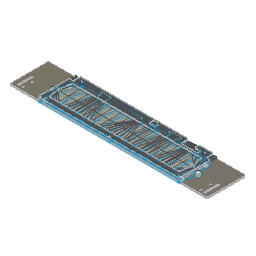
slidrr-housing (Autodesk Fusion 360 design; units mm, degrees)
part number: 2026-08-23-00-43-32-285
Autodesk Fusion 360 part; units mm, degrees
note: some values were not read from the file. Chosen so that the rebuilt part matches the saved one: which bodies a step acts on.
(part 1 of 2)
sketch "Primitive 1 (Outline + Screw Holes)" plane through (0, 0, 0) normal (0, 1, 0) x (1, 0, 0)
  line L0 (3, 0) -> (496.9999, 0)
  line L1 (499.9999, 3) -> (499.9999, 133.475)
  line L2 (496.9999, 136.475) -> (3, 136.475)
  line L3 (0, 133.475) -> (0, 3)
  arc A0 (499.9999, 133.475) -> (496.9999, 136.475) centre (496.9999, 133.475) ccw
  arc A1 (496.9999, 0) -> (499.9999, 3) centre (496.9999, 3) ccw
  arc A2 (0, 3) -> (3, 0) centre (3, 3) ccw
  arc A3 (3, 136.475) -> (0, 133.475) centre (3, 133.475) ccw
  circle A4 centre (495.2019, 4.225) radius 1.5
  circle A5 centre (250.0019, 4.225) radius 1.5
  circle A6 centre (5.0019, 4.225) radius 1.5
  circle A7 centre (6.475, 60.375) radius 1.5
  circle A8 centre (493.525, 60.375) radius 1.5
  circle A9 centre (469.2019, 123.225) radius 1.5
  circle A10 centre (31.0019, 123.225) radius 1.5
  circle A11 centre (250.0019, 117.225) radius 1.5
  point P0 (0, 136.475)
  dimension "d1" = 136.475
  dimension "d2" = 3
  dimension "d3" = 3
  dimension "d4" = 3
  dimension "d5" = 3
  dimension "d7" = 3
  dimension "d8" = 3
  dimension "d9" = 3
  dimension "d10" = 3
  dimension "d11" = 3
  constraint horizontal L0
  constraint vertical L1
  constraint horizontal L2
  constraint vertical L3
  constraint tangent L1 A0
  constraint tangent L2 A0
  constraint tangent L0 A1
  constraint tangent L1 A1
  constraint equal A0 A1
  constraint coincident origin L0
  constraint coincident origin L3
  constraint tangent L0 A2
  constraint tangent L3 A2
  constraint equal A0 A2
  constraint coincident P0 L2
  constraint coincident P0 L3
  constraint tangent L2 A3
  constraint tangent L3 A3
  constraint equal A0 A3
  measures "d1" distance of origin P0
  measures "d2" radius of A0
  measures "d3" diameter of A4
  measures "d4" diameter of A5
  measures "d5" diameter of A6
  measures "d7" diameter of A7
  measures "d8" diameter of A8
  measures "d9" diameter of A9
  measures "d10" diameter of A10
  measures "d11" diameter of A11
other "Base Mesh Feature3"
other "Modify13"
other "Modify14"
sketch "Midplate LGP" plane through (0, 0, 0) normal (0, 1, 0) x (1, 0, 0)
  line L0 (306.25, 19.35) -> (306.25, 101.35)
  arc A0 (0, 3) -> (3, 0) centre (3, 3) ccw
  line L1 (128, 106) -> (106, 106)
  line L2 (300, 128) -> (300, 118)
  line L3 (103.25, 19.35) -> (103.25, 101.35)
  arc A1 (434.5275, 124) -> (437.5275, 121) centre (437.5275, 124) ccw
  line L4 (3, 0) -> (497.0008, 0)
  line L5 (394, 136.475) -> (17, 136.475)
  line L6 (422.25, 19.35) -> (422.25, 101.35)
  line L7 (454.75, 19.35) -> (454.75, 101.35)
  line L8 (281, 131) -> (297, 131)
  arc A2 (98, 130) -> (95, 127) centre (98, 127) ccw
  arc A3 (297, 115) -> (300, 118) centre (297, 118) ccw
  arc A4 (300, 128) -> (297, 131) centre (297, 128) ccw
  line L9 (338.75, 19.35) -> (338.75, 101.35)
  line L10 (19.75, 19.35) -> (19.75, 101.35)
  arc A5 (486.0019, 133.475) -> (483.0019, 136.475) centre (483.0019, 133.475) ccw
  line L11 (434.5275, 133.475) -> (434.5275, 124)
  line L12 (278, 118) -> (278, 128)
  circle A6 centre (5.0019, 4.225) radius 1.5
  line L13 (48.75, 19.35) -> (48.75, 101.35)
  line L14 (397, 112) -> (397, 133.475)
  circle A7 centre (469.2019, 123.225) radius 1.5
  line L15 (135.75, 19.35) -> (135.75, 101.35)
  line L16 (251.75, 19.35) -> (251.75, 101.35)
  line L17 (486.0019, 114) -> (486.0019, 133.475)
  line L18 (374, 110) -> (374, 121)
  line L19 (100, 123) -> (98, 123)
  arc A8 (377, 124) -> (374, 121) centre (377, 121) ccw
  line L20 (132.25, 19.35) -> (132.25, 101.35)
  line L21 (309.75, 19.35) -> (309.75, 101.35)
  line L22 (219.25, 19.35) -> (219.25, 101.35)
  line L23 (95, 126) -> (95, 127)
  circle A9 centre (495.2019, 4.225) radius 1.5
  line L24 (193.75, 19.35) -> (193.75, 101.35)
  line L25 (437.5275, 121) -> (454, 121)
  line L26 (14, 114) -> (14, 133.475)
  line L27 (335.25, 19.35) -> (335.25, 101.35)
  arc A10 (486.0019, 114) -> (489.0019, 111) centre (489.0019, 114) ccw
  circle A11 centre (250.0019, 4.225) radius 1.5
  line L28 (222.75, 19.35) -> (222.75, 101.35)
  line L29 (77.75, 19.35) -> (77.75, 101.35)
  line L30 (451.25, 19.35) -> (451.25, 101.35)
  line L31 (457, 118) -> (457, 112)
  arc A12 (371, 107) -> (374, 110) centre (371, 110) ccw
  arc A13 (377, 124) -> (380, 127) centre (377, 127) ccw
  arc A14 (103, 109) -> (106, 106) centre (106, 109) ccw
  arc A15 (499.9999, 108) -> (496.9999, 111) centre (496.9999, 108) ccw
  circle A16 centre (6.475, 60.35) radius 1.5
  line L32 (297, 115) -> (281, 115)
  arc A17 (340, 131) -> (337, 128) centre (340, 128) ccw
  line L33 (367.75, 19.35) -> (367.75, 101.35)
  arc A18 (131, 127) -> (128, 130) centre (128, 127) ccw
  line L34 (248.25, 19.35) -> (248.25, 101.35)
  line L35 (496.9999, 111) -> (489.0019, 111)
  arc A19 (457, 118) -> (454, 121) centre (454, 118) ccw
  line L36 (74.25, 19.35) -> (74.25, 101.35)
  line L37 (0, 108) -> (0, 3)
  line L38 (371, 107) -> (351, 107)
  line L39 (454, 109) -> (400, 109)
  line L40 (364.25, 19.35) -> (364.25, 101.35)
  line L41 (451.25, 19.35) -> (439.25, 19.35) construction
  line L42 (425.75, 19.35) -> (425.75, 101.35)
  line L43 (190.25, 19.35) -> (190.25, 101.35)
  arc A20 (437.5275, 136.475) -> (434.5275, 133.475) centre (437.5275, 133.475) ccw
  arc A21 (380, 128) -> (377, 131) centre (377, 128) ccw
  arc A22 (11, 111) -> (14, 114) centre (11, 114) ccw
  arc A23 (17, 136.475) -> (14, 133.475) centre (17, 133.475) ccw
  line L44 (106.75, 19.35) -> (106.75, 101.35)
  line L45 (164.75, 19.35) -> (164.75, 101.35)
  line L46 (483.0019, 136.475) -> (437.5275, 136.475)
  line L47 (396.75, 19.35) -> (396.75, 101.35)
  arc A24 (128, 106) -> (131, 109) centre (128, 109) ccw
  arc A25 (95, 126) -> (98, 123) centre (98, 126) ccw
  arc A26 (278, 118) -> (281, 115) centre (281, 118) ccw
  line L48 (337, 127) -> (337, 128)
  line L49 (499.9999, 2.9991) -> (499.9999, 108)
  arc A27 (397, 112) -> (400, 109) centre (400, 112) ccw
  line L50 (131, 123) -> (131, 109)
  arc A28 (337, 127) -> (340, 124) centre (340, 127) ccw
  line L51 (340, 131) -> (377, 131)
  circle A29 centre (6.475, 60.375) radius 1.5
  line L52 (131, 123) -> (131, 127)
  arc A30 (3, 111) -> (0, 108) centre (3, 108) ccw
  line L53 (380, 128) -> (380, 127)
  arc A31 (348, 121) -> (345, 124) centre (345, 121) ccw
  arc A32 (454, 109) -> (457, 112) centre (454, 112) ccw
  circle A33 centre (31, 123.225) radius 1.5
  line L54 (280.75, 19.35) -> (280.75, 101.35)
  line L55 (345, 124) -> (340, 124)
  arc A34 (281, 131) -> (278, 128) centre (281, 128) ccw
  line L56 (45.25, 19.35) -> (45.25, 101.35)
  arc A35 (103, 120) -> (100, 123) centre (100, 120) ccw
  arc A36 (348, 110) -> (351, 107) centre (351, 110) ccw
  line L57 (348, 110) -> (348, 121)
  arc A37 (397, 133.475) -> (394, 136.475) centre (394, 133.475) ccw
  circle A38 centre (31.0019, 123.225) radius 1.5
  line L58 (3, 111) -> (11, 111)
  line L59 (393.25, 19.35) -> (393.25, 101.35)
  line L60 (480.25, 101.35) -> (480.25, 19.35)
  line L61 (103, 109) -> (103, 120)
  line L62 (128, 130) -> (98, 130)
  line L63 (161.25, 19.35) -> (161.25, 101.35)
  circle A39 centre (493.525, 60.375) radius 1.5
  line L64 (277.25, 19.35) -> (277.25, 101.35)
  circle A40 centre (250.0019, 117.225) radius 1.5
  arc A41 (497.0008, 0) -> (499.9999, 2.9991) centre (497.0008, 2.9991) ccw
  line L65 (454.75, 19.35) -> (457.8282, 10.8928)
  line L66 (451.25, 19.35) -> (448.1718, 10.8928)
  line L67 (451.25, 19.35) -> (441.1364, 19.35) construction
  line L68 (457.8282, 10.8928) -> (448.1718, 10.8928)
  line L69 (480.25, 19.35) -> (477.1718, 10.8928)
  line L70 (480.25, 19.35) -> (471.25, 19.35) construction
  line L71 (477.1718, 10.8928) -> (457.8282, 10.8928)
  line L72 (448.1718, 10.8928) -> (428.8282, 10.8928)
  line L73 (425.75, 19.35) -> (428.8282, 10.8928)
  line L74 (428.8282, 10.8928) -> (419.1718, 10.8928)
  line L75 (422.25, 19.35) -> (419.1718, 10.8928)
  line L76 (419.1718, 10.8928) -> (399.8282, 10.8928)
  line L77 (396.75, 19.35) -> (399.8282, 10.8928)
  line L78 (399.8282, 10.8928) -> (390.1718, 10.8928)
  line L79 (393.25, 19.35) -> (390.1718, 10.8928)
  line L80 (390.1718, 10.8928) -> (370.8282, 10.8928)
  line L81 (367.75, 19.35) -> (370.8282, 10.8928)
  line L82 (370.8282, 10.8928) -> (361.1718, 10.8928)
  line L83 (364.25, 19.35) -> (361.1718, 10.8928)
  line L84 (361.1718, 10.8928) -> (341.8282, 10.8928)
  line L85 (338.75, 19.35) -> (341.8282, 10.8928)
  line L86 (341.8282, 10.8928) -> (332.1718, 10.8928)
  line L87 (335.25, 19.35) -> (332.1718, 10.8928)
  line L88 (332.1718, 10.8928) -> (312.8282, 10.8928)
  line L89 (309.75, 19.35) -> (312.8282, 10.8928)
  line L90 (312.8282, 10.8928) -> (303.1718, 10.8928)
  line L91 (306.25, 19.35) -> (303.1718, 10.8928)
  line L92 (303.1718, 10.8928) -> (283.8282, 10.8928)
  line L93 (280.75, 19.35) -> (283.8282, 10.8928)
  line L94 (283.8282, 10.8928) -> (274.1718, 10.8928)
  line L95 (277.25, 19.35) -> (274.1718, 10.8928)
  line L96 (274.1718, 10.8928) -> (254.8282, 10.8928)
  line L97 (251.75, 19.35) -> (254.8282, 10.8928)
  line L98 (254.8282, 10.8928) -> (245.1718, 10.8928)
  line L99 (248.25, 19.35) -> (245.1718, 10.8928)
  line L100 (245.1718, 10.8928) -> (225.8282, 10.8928)
  line L101 (222.75, 19.35) -> (225.8282, 10.8928)
  line L102 (225.8282, 10.8928) -> (216.1718, 10.8928)
  line L103 (219.25, 19.35) -> (216.1718, 10.8928)
  line L104 (216.1718, 10.8928) -> (196.8282, 10.8928)
  line L105 (193.75, 19.35) -> (196.8282, 10.8928)
  line L106 (196.8282, 10.8928) -> (187.1718, 10.8928)
  line L107 (190.25, 19.35) -> (187.1718, 10.8928)
  line L108 (187.1718, 10.8928) -> (167.8282, 10.8928)
  line L109 (164.75, 19.35) -> (167.8282, 10.8928)
  line L110 (167.8282, 10.8928) -> (158.1718, 10.8928)
  line L111 (161.25, 19.35) -> (158.1718, 10.8928)
  line L112 (158.1718, 10.8928) -> (138.8282, 10.8928)
  line L113 (135.75, 19.35) -> (138.8282, 10.8928)
  line L114 (138.8282, 10.8928) -> (129.1718, 10.8928)
  line L115 (132.25, 19.35) -> (129.1718, 10.8928)
  line L116 (129.1718, 10.8928) -> (109.8282, 10.8928)
  line L117 (106.75, 19.35) -> (109.8282, 10.8928)
  line L118 (109.8282, 10.8928) -> (100.1718, 10.8928)
  line L119 (103.25, 19.35) -> (100.1718, 10.8928)
  line L120 (100.1718, 10.8928) -> (80.8282, 10.8928)
  line L121 (77.75, 19.35) -> (80.8282, 10.8928)
  line L122 (80.8282, 10.8928) -> (71.1718, 10.8928)
  line L123 (74.25, 19.35) -> (71.1718, 10.8928)
  line L124 (71.1718, 10.8928) -> (51.8282, 10.8928)
  line L125 (48.75, 19.35) -> (51.8282, 10.8928)
  line L126 (51.8282, 10.8928) -> (42.1718, 10.8928)
  line L127 (45.25, 19.35) -> (42.1718, 10.8928)
  line L128 (42.1718, 10.8928) -> (22.8282, 10.8928)
  line L129 (19.75, 19.35) -> (22.8282, 10.8928)
  point P0 (0, 136.475)
  dimension "d44" = 136.475
  dimension "d45" = 3
  dimension "d46" = 3
  dimension "d47" = 3
  dimension "d48" = 3
  dimension "d49" = 3
  dimension "d50" = 3
  dimension "d51" = 3
  dimension "d52" = 3
  dimension "d53" = 3
  dimension "d54" = 3
  dimension "d55" = 3
  dimension "d56" = 3
  dimension "d57" = 3
  dimension "d63" = 9
  dimension "d65" = 70
  dimension "d66" = 70
  dimension "d69" = -435
  dimension "d70" = 0
  constraint horizontal L4
  constraint vertical L49
  constraint horizontal L46
  constraint vertical L37
  constraint tangent L4 A41
  constraint tangent L49 A41
  constraint coincident origin L4
  constraint coincident origin L37
  constraint tangent A0 L4
  constraint tangent A0 L37
  constraint coincident P0 L5
  constraint coincident P0 L37
  constraint perpendicular L11 L46
  constraint perpendicular L11 L25
  constraint perpendicular L25 L31
  constraint perpendicular L31 L39
  constraint perpendicular L5 L14
  constraint perpendicular L5 L53
  constraint perpendicular L38 L53
  constraint perpendicular L38 L57
  constraint perpendicular L55 L57
  constraint perpendicular L48 L55
  constraint perpendicular L51 L53
  constraint perpendicular L18 L38
  constraint horizontal L8
  constraint perpendicular L2 L8
  constraint perpendicular L2 L32
  constraint perpendicular L8 L12
  constraint perpendicular L8 L50
  constraint perpendicular L1 L50
  constraint perpendicular L8 L61
  constraint perpendicular L19 L50
  constraint perpendicular L19 L23
  constraint parallel L50 L52
  constraint perpendicular L52 L62
  constraint perpendicular L37 L58
  constraint perpendicular L5 L26
  constraint collinear L5 L46
  constraint tangent A31 L57
  constraint tangent A31 L55
  constraint tangent A28 L55
  constraint tangent L48 A28
  constraint equal A28 A31
  constraint tangent A17 L48
  constraint tangent A17 L51
  constraint equal A17 A31
  constraint tangent A21 L53
  constraint tangent A21 L51
  constraint equal A21 A31
  constraint tangent A13 L53
  constraint equal A13 A31
  constraint equal A8 A31
  constraint coincident A8.start A13.start
  constraint tangent L18 A12
  constraint tangent A12 L38
  constraint equal A12 A31
  constraint tangent L38 A36
  constraint tangent A36 L57
  constraint tangent L8 A34
  constraint tangent L12 A34
  constraint tangent L32 A26
  constraint tangent L12 A26
  constraint equal A26 A34
  constraint tangent L2 A3
  constraint tangent A3 L32
  constraint equal A3 A34
  constraint tangent L8 A4
  constraint tangent L2 A4
  constraint equal A4 A34
  constraint tangent A24 L50
  constraint tangent L1 A24
  constraint equal A24 A34
  constraint tangent L1 A14
  constraint tangent A14 L61
  constraint equal A14 A34
  constraint tangent A35 L61
  constraint tangent L19 A35
  constraint equal A34 A35
  constraint tangent L19 A25
  constraint tangent L23 A25
  constraint equal A25 A34
  constraint tangent A2 L23
  constraint tangent A2 L62
  constraint equal A2 A34
  constraint tangent A18 L52
  constraint tangent A18 L62
  constraint equal A18 A34
  constraint tangent L26 A23
  constraint tangent L5 A23
  constraint tangent A22 L58
  constraint tangent L26 A22
  constraint equal A22 A23
  constraint tangent A30 L58
  constraint tangent L37 A30
  constraint equal A23 A30
  constraint tangent L39 A27
  constraint tangent L14 A27
  constraint tangent L14 A37
  constraint tangent L5 A37
  constraint equal A27 A37
  constraint tangent A1 L11
  constraint tangent A1 L25
  constraint equal A1 A27
  constraint tangent L11 A20
  constraint tangent A20 L46
  constraint equal A20 A27
  constraint tangent L31 A32
  constraint tangent L39 A32
  constraint equal A27 A32
  constraint tangent L25 A19
  constraint tangent L31 A19
  constraint equal A19 A27
  constraint tangent A5 L17
  constraint tangent A5 L46
  constraint equal A5 A27
  constraint tangent A10 L35
  constraint tangent L17 A10
  constraint equal A10 A27
  constraint tangent A15 L35
  constraint tangent A15 L49
  constraint equal A15 A27
  constraint horizontal L41
  constraint horizontal L67
  constraint horizontal L68
  constraint horizontal L70
  constraint parallel L68 L71
  measures "d44" distance of origin P0
  measures "d45" diameter of A9
  measures "d46" diameter of A11
  measures "d47" diameter of A6
  measures "d48" diameter of A29
  measures "d49" diameter of A39
  measures "d50" diameter of A7
  measures "d51" diameter of A38
  measures "d52" diameter of A40
  measures "d53" radius of A31
  measures "d54" radius of A36
  measures "d55" radius of A34
  measures "d56" radius of A23
  measures "d57" radius of A27
  measures "d63" distance of L7.start L65.end
  measures "d65" angle of L66 L67
  measures "d66" angle of L69 L70
sketch "Top Shroud" plane through (0, 0, 0) normal (0, 1, 0) x (1, 0, 0)
  line L0 (3, 111) -> (11, 111)
  circle A0 centre (31.0019, 123.225) radius 1.5
  line L1 (394, 136.475) -> (17, 136.475)
  line L2 (499.9999, 2.9991) -> (499.9999, 108)
  arc A1 (3, 111) -> (0, 108) centre (3, 108) ccw
  line L3 (0, 108) -> (0, 3)
  circle A2 centre (250.0019, 117.225) radius 1.5
  arc A3 (17, 136.475) -> (14, 133.475) centre (17, 133.475) ccw
  line L4 (14, 114) -> (14, 133.475)
  circle A4 centre (31, 123.225) radius 1.5
  arc A5 (11, 111) -> (14, 114) centre (11, 114) ccw
  line L5 (451.25, 19.35) -> (439.25, 19.35) construction
  line L6 (3, 0) -> (497.0008, 0)
  line L7 (397, 112) -> (397, 133.475)
  arc A6 (397, 112) -> (400, 109) centre (400, 112) ccw
  line L8 (496.9999, 111) -> (489.0019, 111)
  circle A7 centre (250.0019, 4.225) radius 1.5
  line L9 (451.25, 19.35) -> (441.1364, 19.35) construction
  arc A8 (486.0019, 133.475) -> (483.0019, 136.475) centre (483.0019, 133.475) ccw
  circle A9 centre (6.475, 60.375) radius 1.5
  circle A10 centre (5.0019, 4.225) radius 1.5
  arc A11 (397, 133.475) -> (394, 136.475) centre (394, 133.475) ccw
  arc A12 (434.5275, 124) -> (437.5275, 121) centre (437.5275, 124) ccw
  circle A13 centre (6.475, 60.35) radius 1.5
  arc A14 (457, 118) -> (454, 121) centre (454, 118) ccw
  line L10 (480.25, 19.35) -> (471.25, 19.35) construction
  line L11 (434.5275, 133.475) -> (434.5275, 124)
  arc A15 (0, 3) -> (3, 0) centre (3, 3) ccw
  arc A16 (486.0019, 114) -> (489.0019, 111) centre (489.0019, 114) ccw
  arc A17 (437.5275, 136.475) -> (434.5275, 133.475) centre (437.5275, 133.475) ccw
  arc A18 (499.9999, 108) -> (496.9999, 111) centre (496.9999, 108) ccw
  line L12 (486.0019, 114) -> (486.0019, 133.475)
  line L13 (483.0019, 136.475) -> (437.5275, 136.475)
  line L14 (437.5275, 121) -> (454, 121)
  line L15 (454, 109) -> (400, 109)
  line L16 (457, 118) -> (457, 112)
  circle A19 centre (469.2019, 123.225) radius 1.5
  arc A20 (454, 109) -> (457, 112) centre (454, 112) ccw
  circle A21 centre (493.525, 60.375) radius 1.5
  arc A22 (497.0008, 0) -> (499.9999, 2.9991) centre (497.0008, 2.9991) ccw
  circle A23 centre (495.2019, 4.225) radius 1.5
  line L17 (21.4282, 101.35) -> (478.5718, 101.35)
  line L18 (21.4282, 19.35) -> (478.5718, 19.35)
  line L19 (480.5414, 99.6973) -> (487.1732, 62.0865)
  line L20 (480.25, 101.35) -> (521.8825, 101.35) construction
  line L21 (487.1732, 58.6135) -> (480.5414, 21.0027)
  line L22 (19.4586, 99.6973) -> (12.888, 62.4338)
  line L23 (19.75, 101.35) -> (-21.8825, 101.35) construction
  line L24 (12.888, 58.2662) -> (19.4586, 21.0027)
  arc A24 (12.888, 62.4338) -> (12.888, 58.2662) centre (24.7057, 60.35) ccw
  arc A25 (487.1732, 58.6135) -> (487.1732, 62.0865) centre (477.3251, 60.35) ccw
  arc A26 (480.5414, 99.6973) -> (478.5718, 101.35) centre (478.5718, 99.35) ccw
  arc A27 (478.5718, 19.35) -> (480.5414, 21.0027) centre (478.5718, 21.35) ccw
  arc A28 (19.4586, 21.0027) -> (21.4282, 19.35) centre (21.4282, 21.35) ccw
  arc A29 (21.4282, 101.35) -> (19.4586, 99.6973) centre (21.4282, 99.35) ccw
  arc A30 (278, 118) -> (281, 115) centre (281, 118) ccw
  line L25 (278, 118) -> (278, 128)
  arc A31 (281, 131) -> (278, 128) centre (281, 128) ccw
  line L26 (281, 131) -> (297, 131)
  arc A32 (300, 128) -> (297, 131) centre (297, 128) ccw
  line L27 (300, 128) -> (300, 118)
  arc A33 (297, 115) -> (300, 118) centre (297, 118) ccw
  line L28 (297, 115) -> (281, 115)
  point P0 (0, 136.475)
  dimension "d85" = 136.475
  dimension "d86" = 3
  dimension "d87" = 3
  dimension "d88" = 3
  dimension "d89" = 3
  dimension "d90" = 3
  dimension "d91" = 3
  dimension "d92" = 3
  dimension "d93" = 3
  dimension "d97" = 3
  dimension "d98" = 3
  dimension "d102" = 80
  dimension "d103" = 80
  dimension "d104" = 12
  dimension "d105" = 10
  dimension "d106" = 2
  dimension "d107" = 2
  dimension "d108" = 2
  dimension "d109" = 2
  dimension "d110" = 3
  constraint horizontal L6
  constraint vertical L2
  constraint horizontal L13
  constraint vertical L3
  constraint tangent L6 A22
  constraint tangent L2 A22
  constraint coincident origin L6
  constraint coincident origin L3
  constraint tangent L6 A15
  constraint tangent L3 A15
  constraint coincident P0 L1
  constraint coincident P0 L3
  constraint perpendicular L11 L13
  constraint perpendicular L11 L14
  constraint perpendicular L14 L16
  constraint perpendicular L15 L16
  constraint perpendicular L1 L7
  constraint perpendicular L0 L3
  constraint perpendicular L1 L4
  constraint collinear L1 L13
  constraint tangent A3 L4
  constraint tangent L1 A3
  constraint tangent L0 A5
  constraint tangent L4 A5
  constraint equal A3 A5
  constraint tangent L0 A1
  constraint tangent A1 L3
  constraint equal A1 A3
  constraint tangent A6 L15
  constraint tangent L7 A6
  constraint tangent L7 A11
  constraint tangent L1 A11
  constraint equal A6 A11
  constraint tangent A12 L11
  constraint tangent A12 L14
  constraint equal A6 A12
  constraint tangent L11 A17
  constraint tangent A17 L13
  constraint equal A6 A17
  constraint tangent L16 A20
  constraint tangent L15 A20
  constraint equal A6 A20
  constraint tangent A14 L14
  constraint tangent A14 L16
  constraint equal A6 A14
  constraint tangent A8 L12
  constraint tangent A8 L13
  constraint equal A6 A8
  constraint tangent L8 A16
  constraint tangent A16 L12
  constraint equal A6 A16
  constraint tangent L8 A18
  constraint tangent L2 A18
  constraint equal A6 A18
  constraint horizontal L5
  constraint horizontal L9
  constraint horizontal L10
  constraint horizontal L20
  constraint horizontal L23
  constraint tangent L22 A24
  constraint tangent L24 A24
  constraint tangent L19 A25
  constraint tangent L21 A25
  constraint coincident L20.start L19
  constraint coincident L20.start L17
  constraint tangent L19 A26
  constraint tangent L17 A26
  constraint coincident L10.start L18
  constraint coincident L10.start L21
  constraint tangent L18 A27
  constraint tangent L21 A27
  constraint tangent L18 A28
  constraint tangent L24 A28
  constraint coincident L23.start L17
  constraint coincident L23.start L22
  constraint tangent L17 A29
  constraint tangent L22 A29
  constraint horizontal L26
  constraint perpendicular L26 L27
  constraint perpendicular L27 L28
  constraint perpendicular L25 L26
  constraint tangent A31 L26
  constraint tangent L25 A31
  constraint tangent A30 L28
  constraint tangent A30 L25
  constraint equal A30 A31
  constraint tangent L27 A33
  constraint tangent A33 L28
  constraint equal A31 A33
  constraint tangent L26 A32
  constraint tangent A32 L27
  constraint equal A31 A32
  measures "d85" distance of origin P0
  measures "d86" diameter of A23
  measures "d87" diameter of A7
  measures "d88" diameter of A10
  measures "d89" diameter of A9
  measures "d90" diameter of A21
  measures "d91" diameter of A19
  measures "d92" diameter of A0
  measures "d93" diameter of A2
  measures "d97" radius of A3
  measures "d98" radius of A6
  measures "d102" angle of L19 L20
  measures "d103" angle of L22 L23
  measures "d104" radius of A24
  measures "d105" radius of A25
  measures "d106" radius of A26
  measures "d107" radius of A27
  measures "d108" radius of A28
  measures "d109" radius of A29
  measures "d110" radius of A31
sketch "Base Pieces" plane through (0, 0, 0) normal (0, 1, 0) x (1, 0, 0)
  line L0 (3, 0) -> (696.9999, 0)
  circle A0 centre (350.0019, 117.225) radius 1.5
  line L1 (696.9999, 136.475) -> (3, 136.475)
  circle A1 centre (569.2019, 123.225) radius 1.5
  circle A2 centre (593.525, 60.375) radius 1.5
  circle A3 centre (105.0019, 4.225) radius 1.5
  line L2 (699.9999, 3) -> (699.9999, 133.475)
  arc A4 (0, 3) -> (3, 0) centre (3, 3) ccw
  arc A5 (696.9999, 0) -> (699.9999, 3) centre (696.9999, 3) ccw
  circle A6 centre (350.0019, 4.225) radius 1.5
  circle A7 centre (595.2019, 4.225) radius 1.5
  circle A8 centre (131.0019, 123.225) radius 1.5
  line L3 (0, 133.475) -> (0, 3)
  arc A9 (699.9999, 133.475) -> (696.9999, 136.475) centre (696.9999, 133.475) ccw
  circle A10 centre (106.475, 60.375) radius 1.5
  arc A11 (3, 136.475) -> (0, 133.475) centre (3, 133.475) ccw
  arc A12 (118.3481, 157.7651) -> (114.3481, 161.7651) centre (118.3481, 161.7651) cw
  line L4 (114.3481, 161.7651) -> (114.3481, 173.7651)
  arc A13 (114.3481, 173.7651) -> (118.3481, 177.7651) centre (118.3481, 173.7651) cw
  line L5 (118.3481, 177.7651) -> (277.4892, 177.7651)
  line L6 (476.918, 211.8781) -> (497.4268, 219.1057)
  line L7 (497.4268, 219.1057) -> (494.0066, 209.7088)
  line L8 (494.0066, 209.7088) -> (499.4748, 207.7186)
  line L9 (464.3342, 157.7651) -> (118.3481, 157.7651)
  line L10 (482.3737, 160.7339) -> (476.9056, 162.7242)
  line L11 (473.4854, 153.3273) -> (468.7246, 156.4527)
  arc A14 (468.7246, 156.4527) -> (464.3342, 157.7651) centre (464.3342, 149.7651) ccw
  line L12 (476.9056, 162.7242) -> (473.4854, 153.3273)
  line L13 (499.4748, 207.7186) -> (482.3737, 160.7339)
  circle A15 centre (299.9878, 167.7651) radius 1.5
  circle A16 centre (227.9878, 167.7651) radius 1.5
  line L14 (336.5756, 167.7651) -> (336.5756, 161.7651)
  circle A17 centre (155.9878, 167.7651) radius 1.5
  line L15 (327.5756, 167.7651) -> (327.5756, 161.7651)
  arc A18 (327.5756, 161.7651) -> (328.5756, 160.7651) centre (328.5756, 161.7651) ccw
  line L16 (336.5756, 167.7651) -> (336.5756, 173.7651)
  line L17 (327.5756, 167.7651) -> (327.5756, 173.7651)
  line L18 (335.5756, 174.7651) -> (328.5756, 174.7651)
  arc A19 (336.5756, 173.7651) -> (335.5756, 174.7651) centre (335.5756, 173.7651) ccw
  line L19 (335.5756, 160.7651) -> (328.5756, 160.7651)
  arc A20 (328.5756, 174.7651) -> (327.5756, 173.7651) centre (328.5756, 173.7651) ccw
  arc A21 (335.5756, 160.7651) -> (336.5756, 161.7651) centre (335.5756, 161.7651) ccw
  line L20 (415.5756, 179.7651) -> (408.5756, 179.7651)
  arc A22 (408.5756, 179.7651) -> (407.5756, 178.7651) centre (408.5756, 178.7651) ccw
  line L21 (407.5756, 176.7651) -> (407.5756, 178.7651)
  line L22 (407.5756, 168.7651) -> (407.5756, 166.7651)
  arc A23 (407.5756, 166.7651) -> (408.5756, 165.7651) centre (408.5756, 166.7651) ccw
  line L23 (415.5756, 165.7651) -> (408.5756, 165.7651)
  arc A24 (415.5756, 165.7651) -> (416.5756, 166.7651) centre (415.5756, 166.7651) ccw
  line L24 (416.5756, 168.7651) -> (416.5756, 166.7651)
  line L25 (416.5756, 176.7651) -> (416.5756, 178.7651)
  arc A25 (416.5756, 178.7651) -> (415.5756, 179.7651) centre (415.5756, 178.7651) ccw
  line L26 (408.5756, 175.7651) -> (415.5756, 175.7651)
  line L27 (408.5756, 169.7651) -> (415.5756, 169.7651)
  arc A26 (408.5756, 169.7651) -> (407.5756, 168.7651) centre (408.5756, 168.7651) ccw
  arc A27 (416.5756, 168.7651) -> (415.5756, 169.7651) centre (415.5756, 168.7651) ccw
  arc A28 (415.5756, 175.7651) -> (416.5756, 176.7651) centre (415.5756, 176.7651) ccw
  arc A29 (407.5756, 176.7651) -> (408.5756, 175.7651) centre (408.5756, 176.7651) ccw
  line L28 (114.3481, 161.7651) -> (114.3481, 173.7651)
  line L29 (335.5756, 160.7651) -> (328.5756, 160.7651)
  line L30 (327.5756, 167.7651) -> (327.5756, 161.7651)
  line L31 (464.3342, 157.7651) -> (118.3481, 157.7651)
  line L32 (407.5756, 168.7651) -> (407.5756, 166.7651)
  arc A30 (416.5756, 178.7651) -> (415.5756, 179.7651) centre (415.5756, 178.7651) ccw
  line L33 (415.5756, 165.7651) -> (408.5756, 165.7651)
  arc A31 (407.5756, 176.7651) -> (408.5756, 175.7651) centre (408.5756, 176.7651) ccw
  arc A32 (407.5756, 166.7651) -> (408.5756, 165.7651) centre (408.5756, 166.7651) ccw
  line L34 (415.5756, 179.7651) -> (408.5756, 179.7651)
  line L35 (473.4854, 153.3273) -> (468.7246, 156.4527)
  arc A33 (415.5756, 165.7651) -> (416.5756, 166.7651) centre (415.5756, 166.7651) ccw
  line L36 (408.5756, 175.7651) -> (415.5756, 175.7651)
  line L37 (408.5756, 169.7651) -> (415.5756, 169.7651)
  arc A34 (416.5756, 168.7651) -> (415.5756, 169.7651) centre (415.5756, 168.7651) ccw
  line L38 (327.5756, 167.7651) -> (327.5756, 173.7651)
  line L39 (416.5756, 176.7651) -> (416.5756, 178.7651)
  line L40 (494.0066, 209.7088) -> (499.4748, 207.7186)
  arc A35 (468.7246, 156.4527) -> (464.3342, 157.7651) centre (464.3342, 149.7651) ccw
  line L41 (416.5756, 168.7651) -> (416.5756, 166.7651)
  line L42 (336.5756, 167.7651) -> (336.5756, 161.7651)
  arc A36 (335.5756, 160.7651) -> (336.5756, 161.7651) centre (335.5756, 161.7651) ccw
  arc A37 (336.5756, 173.7651) -> (335.5756, 174.7651) centre (335.5756, 173.7651) ccw
  line L43 (497.4268, 219.1057) -> (494.0066, 209.7088)
  arc A38 (327.5756, 161.7651) -> (328.5756, 160.7651) centre (328.5756, 161.7651) ccw
  arc A39 (118.3481, 157.7651) -> (114.3481, 161.7651) centre (118.3481, 161.7651) cw
  arc A40 (114.3481, 173.7651) -> (118.3481, 177.7651) centre (118.3481, 173.7651) cw
  circle A41 centre (227.9878, 167.7651) radius 1.5
  line L44 (407.5756, 176.7651) -> (407.5756, 178.7651)
  arc A42 (415.5756, 175.7651) -> (416.5756, 176.7651) centre (415.5756, 176.7651) ccw
  arc A43 (408.5756, 179.7651) -> (407.5756, 178.7651) centre (408.5756, 178.7651) ccw
  line L45 (482.3737, 160.7339) -> (476.9056, 162.7242)
  line L46 (476.9056, 162.7242) -> (473.4854, 153.3273)
  circle A44 centre (477.6, 199.7177) radius 2.5
  arc A45 (408.5756, 169.7651) -> (407.5756, 168.7651) centre (408.5756, 168.7651) ccw
  line L47 (476.918, 211.8781) -> (497.4268, 219.1057)
  line L48 (335.5756, 174.7651) -> (328.5756, 174.7651)
  circle A46 centre (299.9878, 167.7651) radius 1.5
  line L49 (499.4748, 207.7186) -> (482.3737, 160.7339)
  arc A47 (328.5756, 174.7651) -> (327.5756, 173.7651) centre (328.5756, 173.7651) ccw
  line L50 (336.5756, 167.7651) -> (336.5756, 173.7651)
  circle A48 centre (155.9878, 167.7651) radius 1.5
  line L51 (103.5756, 203.7651) -> (103.5756, 205.7651)
  arc A49 (42.4266, 216.0775) -> (46.817, 214.7651) centre (46.817, 222.7651) ccw
  arc A50 (103.5756, 195.7651) -> (102.5756, 196.7651) centre (102.5756, 195.7651) ccw
  line L52 (95.5756, 206.7651) -> (102.5756, 206.7651)
  arc A51 (183.5756, 210.7651) -> (182.5756, 211.7651) centre (182.5756, 210.7651) ccw
  line L53 (94.5756, 195.7651) -> (94.5756, 193.7651)
  arc A52 (94.5756, 203.7651) -> (95.5756, 202.7651) centre (95.5756, 203.7651) ccw
  line L54 (13.7244, 153.4245) -> (17.1446, 162.8214)
  arc A53 (183.5756, 210.7651) -> (182.5756, 211.7651) centre (182.5756, 210.7651) ccw
  line L55 (13.7244, 153.4245) -> (17.1446, 162.8214)
  line L56 (17.1446, 162.8214) -> (11.6765, 164.8117)
  line L57 (183.5756, 204.7651) -> (183.5756, 198.7651)
  line L58 (392.8031, 194.7651) -> (233.662, 194.7651)
  arc A54 (233.662, 194.7651) -> (34.2332, 160.6521) centre (233.662, -405.2349) ccw
  line L59 (46.817, 214.7651) -> (392.8031, 214.7651)
  line L60 (34.2332, 160.6521) -> (13.7244, 153.4245)
  line L61 (175.5756, 197.7651) -> (182.5756, 197.7651)
  arc A55 (95.5756, 206.7651) -> (94.5756, 205.7651) centre (95.5756, 205.7651) ccw
  line L62 (94.5756, 203.7651) -> (94.5756, 205.7651)
  line L63 (102.5756, 196.7651) -> (95.5756, 196.7651)
  arc A56 (103.5756, 205.7651) -> (102.5756, 206.7651) centre (102.5756, 205.7651) ccw
  arc A57 (174.5756, 198.7651) -> (175.5756, 197.7651) centre (175.5756, 198.7651) ccw
  line L64 (102.5756, 202.7651) -> (95.5756, 202.7651)
  line L65 (28.7775, 211.7963) -> (34.2456, 209.806)
  line L66 (95.5756, 192.7651) -> (102.5756, 192.7651)
  line L67 (34.2456, 209.806) -> (37.6658, 219.203)
  line L68 (103.5756, 195.7651) -> (103.5756, 193.7651)
  line L69 (102.5756, 196.7651) -> (95.5756, 196.7651)
  circle A58 centre (33.5512, 172.8126) radius 2.5
  arc A59 (102.5756, 202.7651) -> (103.5756, 203.7651) centre (102.5756, 203.7651) ccw
  line L70 (183.5756, 204.7651) -> (183.5756, 210.7651)
  arc A60 (95.5756, 196.7651) -> (94.5756, 195.7651) centre (95.5756, 195.7651) ccw
  arc A61 (175.5756, 211.7651) -> (174.5756, 210.7651) centre (175.5756, 210.7651) ccw
  line L71 (103.5756, 195.7651) -> (103.5756, 193.7651)
  arc A62 (42.4266, 216.0775) -> (46.817, 214.7651) centre (46.817, 222.7651) ccw
  circle A63 centre (211.1634, 204.7651) radius 1.5
  arc A64 (182.5756, 197.7651) -> (183.5756, 198.7651) centre (182.5756, 198.7651) ccw
  line L72 (102.5756, 202.7651) -> (95.5756, 202.7651)
  line L73 (175.5756, 211.7651) -> (182.5756, 211.7651)
  arc A65 (103.5756, 205.7651) -> (102.5756, 206.7651) centre (102.5756, 205.7651) ccw
  arc A66 (94.5756, 203.7651) -> (95.5756, 202.7651) centre (95.5756, 203.7651) ccw
  line L74 (95.5756, 206.7651) -> (102.5756, 206.7651)
  arc A67 (95.5756, 206.7651) -> (94.5756, 205.7651) centre (95.5756, 205.7651) ccw
  arc A68 (95.5756, 196.7651) -> (94.5756, 195.7651) centre (95.5756, 195.7651) ccw
  arc A69 (94.5756, 193.7651) -> (95.5756, 192.7651) centre (95.5756, 193.7651) ccw
  arc A70 (102.5756, 192.7651) -> (103.5756, 193.7651) centre (102.5756, 193.7651) ccw
  arc A71 (103.5756, 195.7651) -> (102.5756, 196.7651) centre (102.5756, 195.7651) ccw
  line L75 (95.5756, 192.7651) -> (102.5756, 192.7651)
  arc A72 (102.5756, 202.7651) -> (103.5756, 203.7651) centre (102.5756, 203.7651) ccw
  line L76 (103.5756, 203.7651) -> (103.5756, 205.7651)
  line L77 (174.5756, 204.7651) -> (174.5756, 198.7651)
  line L78 (34.2332, 160.6521) -> (13.7244, 153.4245)
  arc A73 (392.8031, 214.7651) -> (396.8031, 210.7651) centre (392.8031, 210.7651) cw
  arc A74 (392.8031, 214.7651) -> (396.8031, 210.7651) centre (392.8031, 210.7651) cw
  line L79 (11.6765, 164.8117) -> (28.7775, 211.7963)
  arc A75 (396.8031, 198.7651) -> (392.8031, 194.7651) centre (392.8031, 198.7651) cw
  circle A76 centre (283.1634, 204.7651) radius 1.5
  line L80 (17.1446, 162.8214) -> (11.6765, 164.8117)
  line L81 (392.8031, 194.7651) -> (233.662, 194.7651)
  line L82 (396.8031, 210.7651) -> (396.8031, 198.7651)
  line L83 (11.6765, 164.8117) -> (28.7775, 211.7963)
  line L84 (175.5756, 197.7651) -> (182.5756, 197.7651)
  line L85 (183.5756, 204.7651) -> (183.5756, 210.7651)
  arc A77 (175.5756, 211.7651) -> (174.5756, 210.7651) centre (175.5756, 210.7651) ccw
  line L86 (94.5756, 203.7651) -> (94.5756, 205.7651)
  arc A78 (94.5756, 193.7651) -> (95.5756, 192.7651) centre (95.5756, 193.7651) ccw
  line L87 (174.5756, 204.7651) -> (174.5756, 210.7651)
  line L88 (175.5756, 211.7651) -> (182.5756, 211.7651)
  line L89 (183.5756, 204.7651) -> (183.5756, 198.7651)
  line L90 (37.6658, 219.203) -> (42.4266, 216.0775)
  arc A79 (102.5756, 192.7651) -> (103.5756, 193.7651) centre (102.5756, 193.7651) ccw
  line L91 (34.2456, 209.806) -> (37.6658, 219.203)
  line L92 (28.7775, 211.7963) -> (34.2456, 209.806)
  arc A80 (182.5756, 197.7651) -> (183.5756, 198.7651) centre (182.5756, 198.7651) ccw
  arc A81 (174.5756, 198.7651) -> (175.5756, 197.7651) centre (175.5756, 198.7651) ccw
  line L93 (174.5756, 204.7651) -> (174.5756, 198.7651)
  line L94 (37.6658, 219.203) -> (42.4266, 216.0775)
  line L95 (174.5756, 204.7651) -> (174.5756, 210.7651)
  line L96 (94.5756, 195.7651) -> (94.5756, 193.7651)
  line L97 (680.9505, 10) -> (678.0005, 10)
  line L98 (678.0005, 10) -> (678.0005, 60)
  line L99 (678.0005, 60) -> (680.9505, 60)
  line L100 (683.9505, 60) -> (683.9505, 10)
  line L101 (683.9505, 10) -> (680.9505, 10)
  line L102 (19.0494, 60) -> (16.0494, 60)
  line L103 (16.0494, 60) -> (16.0494, 10)
  line L104 (19.0494, 10) -> (21.9994, 10)
  line L105 (21.9994, 60) -> (19.0494, 60)
  arc A82 (102.5756, 202.7651) -> (103.5756, 203.7651) centre (102.5756, 203.7651) ccw
  arc A83 (415.5756, 175.7651) -> (416.5756, 176.7651) centre (415.5756, 176.7651) ccw
  line L106 (94.5756, 203.7651) -> (94.5756, 205.7651)
  arc A84 (416.5756, 178.7651) -> (415.5756, 179.7651) centre (415.5756, 178.7651) ccw
  line L107 (416.5756, 168.7651) -> (416.5756, 166.7651)
  line L108 (37.6658, 219.203) -> (42.4266, 216.0775)
  arc A85 (175.5756, 211.7651) -> (174.5756, 210.7651) centre (175.5756, 210.7651) ccw
  line L109 (415.5756, 165.7651) -> (408.5756, 165.7651)
  arc A86 (416.5756, 168.7651) -> (415.5756, 169.7651) centre (415.5756, 168.7651) ccw
  line L110 (34.2332, 160.6521) -> (13.7244, 153.4245)
  arc A87 (102.5756, 192.7651) -> (103.5756, 193.7651) centre (102.5756, 193.7651) ccw
  line L111 (34.2456, 209.806) -> (37.6658, 219.203)
  line L112 (407.5756, 176.7651) -> (407.5756, 178.7651)
  line L113 (415.5756, 165.7651) -> (408.5756, 165.7651)
  line L114 (416.5756, 168.7651) -> (416.5756, 166.7651)
  line L115 (13.7244, 153.4245) -> (17.1446, 162.8214)
  arc A88 (415.5756, 175.7651) -> (416.5756, 176.7651) centre (415.5756, 176.7651) ccw
  line L116 (28.7775, 211.7963) -> (34.2456, 209.806)
  line L117 (408.5756, 175.7651) -> (415.5756, 175.7651)
  line L118 (407.5756, 168.7651) -> (407.5756, 166.7651)
  line L119 (174.5756, 204.7651) -> (174.5756, 210.7651)
  line L120 (11.6765, 164.8117) -> (28.7775, 211.7963)
  arc A89 (408.5756, 169.7651) -> (407.5756, 168.7651) centre (408.5756, 168.7651) ccw
  line L121 (94.5756, 195.7651) -> (94.5756, 193.7651)
  line L122 (103.5756, 195.7651) -> (103.5756, 193.7651)
  arc A90 (415.5756, 165.7651) -> (416.5756, 166.7651) centre (415.5756, 166.7651) ccw
  arc A91 (103.5756, 195.7651) -> (102.5756, 196.7651) centre (102.5756, 195.7651) ccw
  line L123 (183.5756, 204.7651) -> (183.5756, 210.7651)
  line L124 (102.5756, 196.7651) -> (95.5756, 196.7651)
  arc A92 (95.5756, 196.7651) -> (94.5756, 195.7651) centre (95.5756, 195.7651) ccw
  arc A93 (103.5756, 205.7651) -> (102.5756, 206.7651) centre (102.5756, 205.7651) ccw
  line L125 (175.5756, 197.7651) -> (182.5756, 197.7651)
  arc A94 (42.4266, 216.0775) -> (46.817, 214.7651) centre (46.817, 222.7651) ccw
  line L126 (17.1446, 162.8214) -> (11.6765, 164.8117)
  line L127 (95.5756, 206.7651) -> (102.5756, 206.7651)
  line L128 (175.5756, 211.7651) -> (182.5756, 211.7651)
  line L129 (407.5756, 176.7651) -> (407.5756, 178.7651)
  line L130 (396.8031, 210.7651) -> (396.8031, 198.7651)
  arc A95 (95.5756, 206.7651) -> (94.5756, 205.7651) centre (95.5756, 205.7651) ccw
  line L131 (183.5756, 204.7651) -> (183.5756, 198.7651)
  arc A96 (174.5756, 198.7651) -> (175.5756, 197.7651) centre (175.5756, 198.7651) ccw
  arc A97 (174.5756, 198.7651) -> (175.5756, 197.7651) centre (175.5756, 198.7651) ccw
  line L132 (37.6658, 219.203) -> (42.4266, 216.0775)
  line L133 (17.1446, 162.8214) -> (11.6765, 164.8117)
  line L134 (102.5756, 196.7651) -> (95.5756, 196.7651)
  line L135 (11.6765, 164.8117) -> (28.7775, 211.7963)
  line L136 (416.5756, 176.7651) -> (416.5756, 178.7651)
  arc A98 (94.5756, 193.7651) -> (95.5756, 192.7651) centre (95.5756, 193.7651) ccw
  line L137 (407.5756, 168.7651) -> (407.5756, 166.7651)
  arc A99 (102.5756, 192.7651) -> (103.5756, 193.7651) centre (102.5756, 193.7651) ccw
  arc A100 (94.5756, 203.7651) -> (95.5756, 202.7651) centre (95.5756, 203.7651) ccw
  line L138 (34.2332, 160.6521) -> (13.7244, 153.4245)
  arc A101 (408.5756, 179.7651) -> (407.5756, 178.7651) centre (408.5756, 178.7651) ccw
  arc A102 (182.5756, 197.7651) -> (183.5756, 198.7651) centre (182.5756, 198.7651) ccw
  line L139 (183.5756, 204.7651) -> (183.5756, 210.7651)
  line L140 (174.5756, 204.7651) -> (174.5756, 210.7651)
  arc A103 (114.3481, 173.7651) -> (118.3481, 177.7651) centre (118.3481, 173.7651) cw
  line L141 (175.5756, 197.7651) -> (182.5756, 197.7651)
  line L142 (416.5756, 176.7651) -> (416.5756, 178.7651)
  line L143 (95.5756, 192.7651) -> (102.5756, 192.7651)
  line L144 (34.2456, 209.806) -> (37.6658, 219.203)
  line L145 (696.9999, 136.475) -> (3, 136.475)
  circle A104 centre (666.05, 13) radius 2.5
  line L146 (680.9505, 60) -> (683.9505, 60)
  line L147 (46.817, 214.7651) -> (392.8031, 214.7651)
  circle A105 centre (666.05, 45) radius 2.5
  line L148 (464.3342, 157.7651) -> (118.3481, 157.7651)
  circle A106 centre (593.525, 60.375) radius 1.5
  line L149 (327.5756, 167.7651) -> (327.5756, 161.7651)
  line L150 (408.5756, 175.7651) -> (415.5756, 175.7651)
  line L151 (21.9994, 10) -> (21.9994, 60)
  arc A107 (408.5756, 169.7651) -> (407.5756, 168.7651) centre (408.5756, 168.7651) ccw
  line L152 (28.7775, 211.7963) -> (34.2456, 209.806)
  line L153 (174.5756, 204.7651) -> (174.5756, 198.7651)
  arc A108 (415.5756, 165.7651) -> (416.5756, 166.7651) centre (415.5756, 166.7651) ccw
  line L154 (94.5756, 203.7651) -> (94.5756, 205.7651)
  arc A109 (335.5756, 160.7651) -> (336.5756, 161.7651) centre (335.5756, 161.7651) ccw
  line L155 (175.5756, 211.7651) -> (182.5756, 211.7651)
  circle A110 centre (44.4959, 202.8827) radius 2.5
  arc A111 (335.5756, 160.7651) -> (336.5756, 161.7651) centre (335.5756, 161.7651) ccw
  line L156 (94.5756, 195.7651) -> (94.5756, 193.7651)
  line L157 (494.0066, 209.7088) -> (499.4748, 207.7186)
  arc A112 (3, 136.475) -> (0, 133.475) centre (3, 133.475) ccw
  line L158 (335.5756, 174.7651) -> (328.5756, 174.7651)
  arc A113 (416.5756, 178.7651) -> (415.5756, 179.7651) centre (415.5756, 178.7651) ccw
  line L159 (335.5756, 160.7651) -> (328.5756, 160.7651)
  line L160 (408.5756, 169.7651) -> (415.5756, 169.7651)
  arc A114 (416.5756, 168.7651) -> (415.5756, 169.7651) centre (415.5756, 168.7651) ccw
  line L161 (13.7244, 153.4245) -> (17.1446, 162.8214)
  line L162 (327.5756, 167.7651) -> (327.5756, 173.7651)
  line L163 (497.4268, 219.1057) -> (494.0066, 209.7088)
  arc A115 (327.5756, 161.7651) -> (328.5756, 160.7651) centre (328.5756, 161.7651) ccw
  line L164 (499.4748, 207.7186) -> (482.3737, 160.7339)
  arc A116 (183.5756, 210.7651) -> (182.5756, 211.7651) centre (182.5756, 210.7651) ccw
  arc A117 (408.5756, 179.7651) -> (407.5756, 178.7651) centre (408.5756, 178.7651) ccw
  line L165 (335.5756, 174.7651) -> (328.5756, 174.7651)
  line L166 (183.5756, 204.7651) -> (183.5756, 198.7651)
  line L167 (476.9056, 162.7242) -> (473.4854, 153.3273)
  line L168 (102.5756, 202.7651) -> (95.5756, 202.7651)
  line L169 (335.5756, 160.7651) -> (328.5756, 160.7651)
  circle A118 centre (355.1634, 204.7651) radius 1.5
  line L170 (174.5756, 204.7651) -> (174.5756, 198.7651)
  arc A119 (468.7246, 156.4527) -> (464.3342, 157.7651) centre (464.3342, 149.7651) ccw
  arc A120 (94.5756, 193.7651) -> (95.5756, 192.7651) centre (95.5756, 193.7651) ccw
  line L171 (336.5756, 167.7651) -> (336.5756, 161.7651)
  arc A121 (102.5756, 202.7651) -> (103.5756, 203.7651) centre (102.5756, 203.7651) ccw
  arc A122 (328.5756, 174.7651) -> (327.5756, 173.7651) centre (328.5756, 173.7651) ccw
  arc A123 (94.5756, 203.7651) -> (95.5756, 202.7651) centre (95.5756, 203.7651) ccw
  arc A124 (175.5756, 211.7651) -> (174.5756, 210.7651) centre (175.5756, 210.7651) ccw
  arc A125 (182.5756, 197.7651) -> (183.5756, 198.7651) centre (182.5756, 198.7651) ccw
  arc A126 (327.5756, 161.7651) -> (328.5756, 160.7651) centre (328.5756, 161.7651) ccw
  line L172 (95.5756, 206.7651) -> (102.5756, 206.7651)
  line L173 (336.5756, 167.7651) -> (336.5756, 173.7651)
  arc A127 (396.8031, 198.7651) -> (392.8031, 194.7651) centre (392.8031, 198.7651) cw
  arc A128 (42.4266, 216.0775) -> (46.817, 214.7651) centre (46.817, 222.7651) ccw
  arc A129 (407.5756, 166.7651) -> (408.5756, 165.7651) centre (408.5756, 166.7651) ccw
  arc A130 (95.5756, 206.7651) -> (94.5756, 205.7651) centre (95.5756, 205.7651) ccw
  circle A131 centre (350.0019, 117.225) radius 1.5
  line L174 (327.5756, 167.7651) -> (327.5756, 173.7651)
  arc A132 (183.5756, 210.7651) -> (182.5756, 211.7651) centre (182.5756, 210.7651) ccw
  line L175 (118.3481, 177.7651) -> (277.4892, 177.7651)
  arc A133 (696.9999, 0) -> (699.9999, 3) centre (696.9999, 3) ccw
  line L176 (464.3342, 157.7651) -> (118.3481, 157.7651)
  line L177 (3, 0) -> (696.9999, 0)
  arc A134 (233.662, 194.7651) -> (34.2332, 160.6521) centre (233.662, -405.2349) ccw
  circle A135 centre (106.475, 60.375) radius 1.5
  arc A136 (277.4892, 177.7651) -> (476.918, 211.8781) centre (277.4892, 777.7651) ccw
  line L178 (0, 133.475) -> (0, 3)
  circle A137 centre (105.0019, 4.225) radius 1.5
  circle A138 centre (350.0019, 4.225) radius 1.5
  line L179 (102.5756, 202.7651) -> (95.5756, 202.7651)
  arc A139 (699.9999, 133.475) -> (696.9999, 136.475) centre (696.9999, 133.475) ccw
  line L180 (699.9999, 3) -> (699.9999, 133.475)
  circle A140 centre (595.2019, 4.225) radius 1.5
  line L181 (476.918, 211.8781) -> (497.4268, 219.1057)
  line L182 (497.4268, 219.1057) -> (494.0066, 209.7088)
  arc A141 (103.5756, 205.7651) -> (102.5756, 206.7651) centre (102.5756, 205.7651) ccw
  line L183 (408.5756, 169.7651) -> (415.5756, 169.7651)
  line L184 (103.5756, 203.7651) -> (103.5756, 205.7651)
  circle A142 centre (33.9499, 13) radius 2.5
  circle A143 centre (299.9878, 167.7651) radius 1.5
  arc A144 (328.5756, 174.7651) -> (327.5756, 173.7651) centre (328.5756, 173.7651) ccw
  arc A145 (95.5756, 196.7651) -> (94.5756, 195.7651) centre (95.5756, 195.7651) ccw
  arc A146 (118.3481, 157.7651) -> (114.3481, 161.7651) centre (118.3481, 161.7651) cw
  line L185 (499.4748, 207.7186) -> (482.3737, 160.7339)
  line L186 (16.0494, 10) -> (19.0494, 10)
  line L187 (473.4854, 153.3273) -> (468.7246, 156.4527)
  arc A147 (336.5756, 173.7651) -> (335.5756, 174.7651) centre (335.5756, 173.7651) ccw
  line L188 (114.3481, 161.7651) -> (114.3481, 173.7651)
  line L189 (473.4854, 153.3273) -> (468.7246, 156.4527)
  circle A148 centre (227.9878, 167.7651) radius 1.5
  line L190 (103.5756, 203.7651) -> (103.5756, 205.7651)
  arc A149 (0, 3) -> (3, 0) centre (3, 3) ccw
  line L191 (476.918, 211.8781) -> (497.4268, 219.1057)
  circle A150 centre (131.0019, 123.225) radius 1.5
  line L192 (415.5756, 179.7651) -> (408.5756, 179.7651)
  line L193 (494.0066, 209.7088) -> (499.4748, 207.7186)
  line L194 (114.3481, 161.7651) -> (114.3481, 173.7651)
  line L195 (482.3737, 160.7339) -> (476.9056, 162.7242)
  line L196 (103.5756, 195.7651) -> (103.5756, 193.7651)
  arc A151 (407.5756, 176.7651) -> (408.5756, 175.7651) centre (408.5756, 176.7651) ccw
  line L197 (336.5756, 167.7651) -> (336.5756, 161.7651)
  arc A152 (103.5756, 195.7651) -> (102.5756, 196.7651) centre (102.5756, 195.7651) ccw
  arc A153 (114.3481, 173.7651) -> (118.3481, 177.7651) centre (118.3481, 173.7651) cw
  line L198 (327.5756, 167.7651) -> (327.5756, 161.7651)
  line L199 (415.5756, 179.7651) -> (408.5756, 179.7651)
  circle A154 centre (155.9878, 167.7651) radius 1.5
  arc A155 (468.7246, 156.4527) -> (464.3342, 157.7651) centre (464.3342, 149.7651) ccw
  line L200 (476.9056, 162.7242) -> (473.4854, 153.3273)
  arc A156 (336.5756, 173.7651) -> (335.5756, 174.7651) centre (335.5756, 173.7651) ccw
  line L201 (336.5756, 167.7651) -> (336.5756, 173.7651)
  line L202 (482.3737, 160.7339) -> (476.9056, 162.7242)
  circle A157 centre (466.6554, 169.6475) radius 2.5
  line L203 (95.5756, 192.7651) -> (102.5756, 192.7651)
  arc A158 (118.3481, 157.7651) -> (114.3481, 161.7651) centre (118.3481, 161.7651) cw
  arc A159 (407.5756, 176.7651) -> (408.5756, 175.7651) centre (408.5756, 176.7651) ccw
  arc A160 (407.5756, 166.7651) -> (408.5756, 165.7651) centre (408.5756, 166.7651) ccw
  circle A161 centre (33.9499, 45) radius 2.5
  circle A162 centre (569.2019, 123.225) radius 1.5
  line L204 (40.6348, -12.1734) -> (386.6208, -12.1734)
  line L205 (112.1658, -49.1734) -> (271.3069, -49.1734)
  arc A163 (96.3933, -24.1734) -> (97.3933, -23.1734) centre (96.3933, -23.1734) ccw
  arc A164 (409.3933, -51.1734) -> (410.3933, -50.1734) centre (409.3933, -50.1734) ccw
  line L206 (88.3933, -23.1734) -> (88.3933, -21.1734)
  arc A165 (410.3933, -48.1734) -> (409.3933, -47.1734) centre (409.3933, -48.1734) ccw
  line L207 (410.3933, -58.1734) -> (410.3933, -60.1734)
  line L208 (31.4836, -7.7355) -> (36.2443, -10.861)
  arc A166 (169.3933, -15.1734) -> (168.3933, -16.1734) centre (169.3933, -16.1734) ccw
  line L209 (409.3933, -61.1734) -> (402.3933, -61.1734)
  arc A167 (410.3933, -58.1734) -> (409.3933, -57.1734) centre (409.3933, -58.1734) ccw
  line L210 (28.0509, -66.2863) -> (7.5421, -73.514)
  line L211 (390.6208, -16.1734) -> (390.6208, -28.1734)
  arc A168 (96.3933, -34.1734) -> (97.3933, -33.1734) centre (96.3933, -33.1734) ccw
  line L212 (28.0633, -17.1324) -> (31.4836, -7.7355)
  line L213 (401.3933, -50.1734) -> (401.3933, -48.1734)
  line L214 (409.3933, -61.1734) -> (402.3933, -61.1734)
  line L215 (410.3933, -58.1734) -> (410.3933, -60.1734)
  line L216 (7.5421, -73.514) -> (10.9623, -64.1171)
  arc A169 (409.3933, -51.1734) -> (410.3933, -50.1734) centre (409.3933, -50.1734) ccw
  line L217 (22.5952, -15.1422) -> (28.0633, -17.1324)
  line L218 (402.3933, -51.1734) -> (409.3933, -51.1734)
  line L219 (401.3933, -58.1734) -> (401.3933, -60.1734)
  line L220 (168.3933, -22.1734) -> (168.3933, -16.1734)
  line L221 (5.4942, -62.1268) -> (22.5952, -15.1422)
  arc A170 (402.3933, -57.1734) -> (401.3933, -58.1734) centre (402.3933, -58.1734) ccw
  line L222 (88.3933, -31.1734) -> (88.3933, -33.1734)
  line L223 (97.3933, -31.1734) -> (97.3933, -33.1734)
  arc A171 (409.3933, -61.1734) -> (410.3933, -60.1734) centre (409.3933, -60.1734) ccw
  arc A172 (97.3933, -31.1734) -> (96.3933, -30.1734) centre (96.3933, -31.1734) ccw
  line L224 (177.3933, -22.1734) -> (177.3933, -16.1734)
  line L225 (96.3933, -30.1734) -> (89.3933, -30.1734)
  arc A173 (89.3933, -30.1734) -> (88.3933, -31.1734) centre (89.3933, -31.1734) ccw
  arc A174 (97.3933, -21.1734) -> (96.3933, -20.1734) centre (96.3933, -21.1734) ccw
  line L226 (169.3933, -29.1734) -> (176.3933, -29.1734)
  arc A175 (36.2443, -10.861) -> (40.6348, -12.1734) centre (40.6348, -4.1734) ccw
  line L227 (10.9623, -64.1171) -> (5.4942, -62.1268)
  line L228 (89.3933, -20.1734) -> (96.3933, -20.1734)
  line L229 (169.3933, -15.1734) -> (176.3933, -15.1734)
  line L230 (401.3933, -50.1734) -> (401.3933, -48.1734)
  line L231 (390.6208, -16.1734) -> (390.6208, -28.1734)
  arc A176 (89.3933, -20.1734) -> (88.3933, -21.1734) centre (89.3933, -21.1734) ccw
  line L232 (177.3933, -22.1734) -> (177.3933, -28.1734)